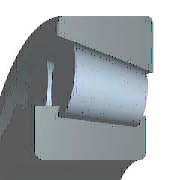
# Autodesk Inventor part: PWTR-0067
Saved by Autodesk Inventor 2021.1 (Build 251245000, 245)
## iProperties
IsCustomPart: 1
Created: 2020-01-21
Part Number: PWTR-0067
Material: Steel, Mild
Description: Taper Roller Bearings Single Row - Precision SKF
Document SubType Name: Modeling
Standard: SKF
Designer: alid
Language: en-US
Size Designation: SKF32004 XC/P5
Categories: <MemberInstance><Categories><Category DisplayName="Shaft Parts" InternalName="7f7aeb1f-a693-4053-b835-cee3144e0d98" Mnemonic="SHFT"><Category DisplayName="Bearings" InternalName="242d30a3-7172-44e6-a363-b0a3d8f1b556" Mnemonic="BRNG"><CategoryParameter DisplayName="Width" InternalName="25fc5f6e-338b-4801-b5ed-8959743e396e" Mnemonic="wdth"/><CategoryParameter DisplayName="Size Designation" InternalName="2c4e891a-c8f4-49ed-a5c1-5131476c6feb" Mnemonic="sizedes"/><CategoryParameter DisplayName="Basic Dynamic Load Rating" InternalName="440972dd-7009-4861-bd45-69ffbb461423" Mnemonic="bdynlrat"/><CategoryParameter DisplayName="Shaft Diameter" InternalName="91302473-2833-4451-a660-c5d4a8d6a031" Mnemonic="shaftdia"/><CategoryParameter DisplayName="Touch Angle" InternalName="aa21a452-7974-4a55-b5cf-1c2972de2aea" Mnemonic="TouchAngle"/><CategoryParameter DisplayName="Outer Diameter" InternalName="d441686c-04bd-4681-b674-94fbc173ec23" Mnemonic="outdia"/><Category DisplayName="Roller Bearings" InternalName="a40a3fd7-d489-4921-9892-cb944902a182" Mnemonic="ROLLBEAR"><CategoryParameter DisplayName="Basic Static Load Rating" InternalName="124ef669-bc53-497e-8b3b-9e9432584ac1" Mnemonic="bstatlrat"/><CategoryParameter DisplayName="Radial Dynamic Load Factor when Fa/Fr &gt; e" InternalName="1feec4eb-3d91-4913-989d-fa96ab069f3d" Mnemonic="raddynfc2"/><CategoryParameter DisplayName="Axial Dynamic Load Factor when Fa/Fr &gt; e" InternalName="200b4357-faba-40fb-9da6-9412c8ddeb78" Mnemonic="axdynfc2"/><CategoryParameter DisplayName="Radius" InternalName="2322b21e-a448-4b16-bf77-0b09a9a1e5fa" Mnemonic="rad"/><CategoryParameter DisplayName="Min. Shaft Diameter" InternalName="27c639de-1f82-42cb-a17a-a84ebe509f1b" Mnemonic="minshaftdia"/><CategoryParameter DisplayName="Limiting Speed Lubrication Grease" InternalName="34ed7782-22cd-44b7-90f2-16a4b10c8234" Mnemonic="lubgrsp"/><CategoryParameter DisplayName="Mass" InternalName="35563771-cdde-4f36-b8ea-a6490dc90073" Mnemonic="mass"/><CategoryParameter DisplayName="Limiting Speed Oil" InternalName="576744bc-a99a-4f12-bf8b-8b83672ef882" Mnemonic="oilspd"/><CategoryParameter DisplayName="Radial Static Load Factor" InternalName="646321f5-f93b-4aec-b962-0341aa1dcfaf" Mnemonic="raddynfc0"/><CategoryParameter DisplayName="Max. Step Fillet Radius" InternalName="890763e8-95b6-457a-9b07-8de657924e40" Mnemonic="maxstprad"/><CategoryParameter DisplayName="Axial Dynamic Load Factor when Fa/Fr &lt;= e" InternalName="b1d498d2-5149-4618-b12c-23a3d5a7c887" Mnemonic="axdynfc1"/><CategoryParameter DisplayName="Radial Dynamic Load Factor when Fa/Fr &lt;= e" InternalName="b75e8b40-fb1d-483d-887b-ce2ffe1b5422" Mnemonic="raddynfc1"/><CategoryParameter DisplayName="Friction Factor" InternalName="ceddb76f-d381-429d-bef5-367584929fdf" Mnemonic="fricfct"/><CategoryParameter DisplayName="Axial Static Load Factor" InternalName="ea413b62-e115-405b-882c-23d570c3be21" Mnemonic="axdynfc0"/><CategoryParameter DisplayName="Limiting Value for Factor Determination" InternalName="f0539972-a230-481a-8ae0-28002199c8fb" Mnemonic="limvalfac"/><CategoryParameter DisplayName="Exponent for Determining Life" InternalName="f80a4cc4-8fb3-4eaa-808e-6f490e608712" Mnemonic="lifeexp"/><CategoryParameter DisplayName="Max. Hub Step Diameter" InternalName="feeea31f-2614-4692-af6e-a054e6e558b2" Mnemonic="maxhubdia"/><Category DisplayName="Tapered Roller Bearings" InternalName="326936b4-87e6-427a-a604-f9fe807308df" Mnemonic="RBTRB"/></Category></Category></Category><Category DisplayName="DataType" InternalName="23b78d0f-2648-40c6-8793-ca6db495c9e8" Mnemonic="DATATYPE"><CategoryParameter DisplayName="DisplayName" InternalName="05415f3d-3907-474b-a020-eb9d644f4cf3" Mnemonic="DISPLAYNAME"/><CategoryParameter DisplayName="Standard" InternalName="0c0a119c-1e12-4c84-803f-101930972f5e" Mnemonic="STANDARD"/><CategoryParameter DisplayName="Description" InternalName="13903e3d-64b1-4950-80da-f627842ea37f" Mnemonic="DESCRIPTION"/><CategoryParameter DisplayName="Designation" InternalName="2675968c-4ce5-49e0-a4f5-552d29089031" Mnemonic="DESIGNATION"/><CategoryParameter DisplayName="Default Row" InternalName="2af9ec52-faaa-4026-b378-f9fa4afca842" Mnemonic="DEFAULTROW"/><CategoryParameter DisplayName="Folder Name" InternalName="3f06958e-8713-4116-9be7-ed6184ecc97b" Mnemonic="FOLDERNAME"/><CategoryParameter DisplayName="Revision Guid" InternalName="45a75005-10b1-4dfc-8d6d-dfe629f0b93c" Mnemonic="REVISIONGUID"/><CategoryParameter DisplayName="FileName" InternalName="8b46a4cc-9585-4fed-90c3-899f57e09a73" Mnemonic="FILENAME"/><CategoryParameter DisplayName="StdsOrg" InternalName="8f5914e1-4693-403f-8ab5-d37768198c9d" Mnemonic="STDSORG"/><CategoryParameter DisplayName="Family Version" InternalName="914462f6-6e19-4b14-ba84-155b9680b1d0" Mnemonic="FAMILYREVISION"/><CategoryParameter DisplayName="Standard Revision" InternalName="91d5a463-65c2-4fde-b823-3b7fea5e8e17" Mnemonic="STANDARDREVISION"/><CategoryParameter DisplayName="Member Revision" InternalName="a65d44b9-392f-4f4f-857b-e4b3d54996fe" Mnemonic="MEMBERREVISION"/><CategoryParameter DisplayName="ClipFormat" InternalName="bc51e27b-3422-4e78-93ef-cec197ddf230" Mnemonic="CLIPFORMAT"/><CategoryParameter DisplayName="Manufacturer" InternalName="cd6c7a72-a28a-4e50-99a9-2c7f4e13e5ad" Mnemonic="MANUFACTURER"/><CategoryParameter DisplayName="InternalName" InternalName="cf1d0246-76d9-4b4a-8305-fa0409afb5c1" Mnemonic="INTERNALNAME"/><CategoryParameter DisplayName="IsMetric" InternalName="e2385c5b-1ea4-4823-96a8-8de651266ec3" Mnemonic="ISMETRIC"/><Category DisplayName="Part" InternalName="c0e0b642-3bcb-4cc8-9e80-f96d35c4afa4" Mnemonic="PART"><CategoryParameter DisplayName="Part Number" InternalName="016b6077-bfbe-49bd-92c9-d8d59c39c941" Mnemonic="PARTNUMBER"/><CategoryParameter DisplayName="Stock Number" InternalName="4dba7c1c-e26c-444e-836c-b08b433409a8" Mnemonic="STOCKNUMBER"/><CategoryParameter DisplayName="Material Key" InternalName="5c9a8adb-dd2b-4535-b97f-0a94a95fe41f" Mnemonic="MATERIALKEY"/><CategoryParameter DisplayName="Material" InternalName="818a152a-d3c3-49ca-80ee-df7d91421b8e" Mnemonic="MATERIAL"/></Category></Category><Category DisplayName="Legacy Map DA" InternalName="924fff40-ddd0-4eff-ad42-30e3774ef79e" Mnemonic="LEGACYMAPDA"><CategoryParameter DisplayName="DACookie" InternalName="316934ee-8fe1-4c7a-9c36-f2d79e1add1a" Mnemonic="DACOOKIE"/></Category><Category DisplayName="LegacyMap" InternalName="cd87c42b-3e48-431e-b5c0-1cbeb14dfe77" Mnemonic="LEGACYMAP"><CategoryParameter DisplayName="unique DA member ID" InternalName="0918ad47-427f-4fed-ae26-24c81c58f590" Mnemonic="DACOOKIE"/><CategoryParameter DisplayName="Merge11 ID" InternalName="0ee8fb18-e2ed-4f39-96f6-1f4b5f50aa71" Mnemonic="MERGE11"/><CategoryParameter DisplayName="unique CC member ID" InternalName="5193edd4-b2b0-4ab4-9d54-de900eee34e0" Mnemonic="CCCOOKIE"/><CategoryParameter DisplayName="Split ID" InternalName="72b5c83c-be7f-45c4-ae51-9160ea6deb26" Mnemonic="SPLIT"/><CategoryParameter DisplayName="MemberID" InternalName="8e5e0294-fc51-4c8f-b3d7-003dc5ed94f6" Mnemonic="MEMBERID"/><CategoryParameter DisplayName="CatalogName" InternalName="d99d1e27-aa94-4de2-af4c-c348882a6f4f" Mnemonic="CATALOGNAME"/><CategoryParameter DisplayName="FamilyNumber" InternalName="e705e1f4-09cb-413e-91f9-551b4188271e" Mnemonic="FAMILYNUMBER"/></Category></Categories><FamilyTemplate Id="N024720"><FamilyTemplateParameters><FamilyTemplateParameter ObjectType="kUserParameterObject" ValueType="xs:integer" Id="1" ObjectReferenceKey="Diam"/><FamilyTemplateParameter ObjectType="kUserParameterObject" ValueType="xs:integer" Id="2" ObjectReferenceKey="DD"/><FamilyTemplateParameter ObjectType="kUserParameterObject" ValueType="xs:double" Id="3" ObjectReferenceKey="B"/><FamilyTemplateParameter ObjectType="kUserParameterObject" ValueType="xs:double" Id="4" ObjectReferenceKey="CC"/><FamilyTemplateParameter ObjectType="kUserParameterObject" ValueType="xs:integer" Id="5" ObjectReferenceKey="ParT"/><FamilyTemplateParameter ObjectType="kUserParameterObject" ValueType="xs:double" Id="6" ObjectReferenceKey="r"/><FamilyTemplateParameter ObjectType="kUserParameterObject" ValueType="xs:integer" Id="8" ObjectReferenceKey="alfa"/><FamilyTemplateParameter ObjectType="kPropertyObject" ValueType="xs:string" Id="100" ObjectReferenceKey="{32853F0F-3444-11d1-9E93-0060B03C1CA6}" SubObjectId="52"/><FamilyTemplateParameter ObjectType="kPropertyObject" ValueType="xs:string" Id="105" ObjectReferenceKey="{32853F0F-3444-11d1-9E93-0060B03C1CA6}" SubObjectId="5"/><FamilyTemplateParameter ObjectType="kPartComponentDefinitionObject" ValueType="xs:string" Id="110" SubObjectId="Material"/></FamilyTemplateParameters></FamilyTemplate><CategoryParameterMap><ParamToTemplateMap><ParamToTemplate CategoryParameter="//CategoryParameter[@InternalName='05415f3d-3907-474b-a020-eb9d644f4cf3']" ConstantValue="SKF- Taper Roller Bearings, Precision"/><ParamToTemplate CategoryParameter="//CategoryParameter[@InternalName='cf1d0246-76d9-4b4a-8305-fa0409afb5c1']" ConstantValue="F84C4950-AFA6-4409-9E95-6F585BEA7148"/><ParamToTemplate CategoryParameter="//CategoryParameter[@InternalName='3f06958e-8713-4116-9be7-ed6184ecc97b']" ConstantValue="SKF - Taper Roller Bearings, Precision"/><ParamToTemplate CategoryParameter="//CategoryParameter[@InternalName='914462f6-6e19-4b14-ba84-155b9680b1d0']" ConstantValue="10"/><ParamToTemplate CategoryParameter="//CategoryParameter[@InternalName='bc51e27b-3422-4e78-93ef-cec197ddf230']" ConstantValue="CF_INVENTOR.STDPARTS"/><ParamToTemplate CategoryParameter="//CategoryParameter[@InternalName='e2385c5b-1ea4-4823-96a8-8de651266ec3']" ConstantValue="true"/><ParamToTemplate CategoryParameter="//CategoryParameter[@InternalName='13903e3d-64b1-4950-80da-f627842ea37f']" ConstantValue="Taper Roller Bearings Single Row - Precision SKF"/><ParamToTemplate CategoryParameter="//CategoryParameter[@InternalName='8f5914e1-4693-403f-8ab5-d37768198c9d']" TemplateParameter="101"/><ParamToTemplate CategoryParameter="//CategoryParameter[@InternalName='0c0a119c-1e12-4c84-803f-101930972f5e']" ConstantValue="SKF"/><ParamToTemplate CategoryParameter="//CategoryParameter[@InternalName='cd6c7a72-a28a-4e50-99a9-2c7f4e13e5ad']" TemplateParameter="104"/><ParamToTemplate CategoryParameter="//CategoryParameter[@InternalName='91d5a463-65c2-4fde-b823-3b7fea5e8e17']" TemplateParameter="103"/><ParamToTemplate CategoryParameter="//CategoryParameter[@InternalName='45a75005-10b1-4dfc-8d6d-dfe629f0b93c']" ConstantValue="35ea33a0-70f2-4056-843a-40b698840a71"/><ParamToTemplate CategoryParameter="//CategoryParameter[@InternalName='2af9ec52-faaa-4026-b378-f9fa4afca842']" ConstantValue="10"/><ParamToTemplate CategoryParameter="//CategoryParameter[@InternalName='8b46a4cc-9585-4fed-90c3-899f57e09a73']" ConstantValue="SKF32004 XC/P5"/><ParamToTemplate CategoryParameter="//CategoryParameter[@InternalName='a65d44b9-392f-4f4f-857b-e4b3d54996fe']" ConstantValue="60633b30-7c0a-4b0a-9e61-588410ecd8ec"/><ParamToTemplate CategoryParameter="//CategoryParameter[@InternalName='124ef669-bc53-497e-8b3b-9e9432584ac1']" ConstantValue="27000"/><ParamToTemplate CategoryParameter="//CategoryParameter[@InternalName='34ed7782-22cd-44b7-90f2-16a4b10c8234']" ConstantValue="8500"/><ParamToTemplate CategoryParameter="//CategoryParameter[@InternalName='ceddb76f-d381-429d-bef5-367584929fdf']" ConstantValue="0.0018"/><ParamToTemplate CategoryParameter="//CategoryParameter[@InternalName='f80a4cc4-8fb3-4eaa-808e-6f490e608712']" ConstantValue="3.33333"/><ParamToTemplate CategoryParameter="//CategoryParameter[@InternalName='27c639de-1f82-42cb-a17a-a84ebe509f1b']" ConstantValue="25"/><ParamToTemplate CategoryParameter="//CategoryParameter[@InternalName='feeea31f-2614-4692-af6e-a054e6e558b2']" ConstantValue="37"/><ParamToTemplate CategoryParameter="//CategoryParameter[@InternalName='890763e8-95b6-457a-9b07-8de657924e40']" ConstantValue="0.6"/><ParamToTemplate CategoryParameter="//CategoryParameter[@InternalName='576744bc-a99a-4f12-bf8b-8b83672ef882']" ConstantValue="12000"/><ParamToTemplate CategoryParameter="//CategoryParameter[@InternalName='f0539972-a230-481a-8ae0-28002199c8fb']" ConstantValue="0.37"/><ParamToTemplate CategoryParameter="//CategoryParameter[@InternalName='646321f5-f93b-4aec-b962-0341aa1dcfaf']" ConstantValue="0.5"/><ParamToTemplate CategoryParameter="//CategoryParameter[@InternalName='ea413b62-e115-405b-882c-23d570c3be21']" ConstantValue="0.9"/><ParamToTemplate CategoryParameter="//CategoryParameter[@InternalName='b75e8b40-fb1d-483d-887b-ce2ffe1b5422']" ConstantValue="1"/><ParamToTemplate CategoryParameter="//CategoryParameter[@InternalName='b1d498d2-5149-4618-b12c-23a3d5a7c887']" ConstantValue="0"/><ParamToTemplate CategoryParameter="//CategoryParameter[@InternalName='2c4e891a-c8f4-49ed-a5c1-5131476c6feb']" ConstantValue="32004 XC/P5"/><ParamToTemplate CategoryParameter="//CategoryParameter[@InternalName='316934ee-8fe1-4c7a-9c36-f2d79e1add1a']" ConstantValue="*ISO~N024720A~SKF 32004 XC/P5*AFN~N024720A~SKF 32004 XC/P5*ANS~N024720A~SKF 32004 XC/P5*"/><ParamToTemplate CategoryParameter="//CategoryParameter[@InternalName='0918ad47-427f-4fed-ae26-24c81c58f590']" ConstantValue="*ISO~N024720A~SKF 32004 XC/P5*AFN~N024720A~SKF 32004 XC/P5*ANS~N024720A~SKF 32004 XC/P5*"/><ParamToTemplate CategoryParameter="//CategoryParameter[@InternalName='0ee8fb18-e2ed-4f39-96f6-1f4b5f50aa71']" ConstantValue="^1FF598A5-DCBF-4D03-99DD-51C67A5B1954^3ADC193E-2142-431A-9EEA-E87C8E0B94A1^36F4839B-D4FF-4949-8334-EE9110708ED8^"/><ParamToTemplate CategoryParameter="//CategoryParameter[@InternalName='25fc5f6e-338b-4801-b5ed-8959743e396e']" TemplateParameter="3"/><ParamToTemplate CategoryParameter="//CategoryParameter[@InternalName='d441686c-04bd-4681-b674-94fbc173ec23']" TemplateParameter="2"/><ParamToTemplate CategoryParameter="//CategoryParameter[@InternalName='2675968c-4ce5-49e0-a4f5-552d29089031']" TemplateParameter="100"/><ParamToTemplate CategoryParameter="//CategoryParameter[@InternalName='91302473-2833-4451-a660-c5d4a8d6a031']" TemplateParameter="1"/><ParamToTemplate CategoryParameter="//CategoryParameter[@InternalName='818a152a-d3c3-49ca-80ee-df7d91421b8e']" TemplateParameter="110"/><ParamToTemplate CategoryParameter="//CategoryParameter[@InternalName='016b6077-bfbe-49bd-92c9-d8d59c39c941']" TemplateParameter="105"/><ParamToTemplate CategoryParameter="//CategoryParameter[@InternalName='2322b21e-a448-4b16-bf77-0b09a9a1e5fa']" TemplateParameter="6"/></ParamToTemplateMap></CategoryParameterMap></MemberInstance>
Density: 7.85 g/cm^3
Appearance: Semi-Polished
Stock Number: SKF32004 XC/P5
Author: alid
Revision Number: A
Autodesk Inventor part; units mm, degrees
ref_plane "WorkPlane4" through (0, 0, 0) normal (0, 0, 1) x (1, 0, 0)
ref_plane "WorkPlane1" through (0, 0, 0) normal (0, 0, 1) x (1, 0, 0)
ref_plane "Work Plane3" through (0, 0, -15) normal (0, 0, 1) x (1, 0, 0)
ref_plane "WorkPlane2" through (0, 0, 15) normal (0, 0, 1) x (1, 0, 0)
sketch "Sketch1" plane through (0, 0, 0) normal (0, 0, 1) x (1, 0, 0)
  point P0 (0, 0)
sketch "Sketch2" plane through (0, 0, 15) normal (0, 0, 1) x (1, 0, 0)
  point P0 (0, 0)
sketch "Sketch3" plane through (0, 0, 0) normal (0, 0, 1) x (1, 0, 0)
  circle A0 centre (0, 0) radius 15.5
  dimension "d2" = 31
extrude "Extrusion1" add sketch "Sketch3" along normal blind 15
sketch "Sketch4" plane through (0, 0, 15) normal (0, 0, 1) x (1, 0, 0)
  circle A0 centre (0, 0) radius 15.5 projected
hole "Hole1" at (0, 0, 15) direction (0, 0, -1) diameter 20 end through all
sketch "Sketch5" plane through (0, 0, 0) normal (1, 0, 0) x (0, 1, 0)
  line L0 (16.471593, 15) -> (14.125, 15)
  line L1 (14.125, 15) -> (14.125, 11.985238)
  line L2 (12.066474, 11.547685) -> (14.125, 11.985238)
  line L3 (12.066474, 11.547685) -> (13.433526, 2.283254)
  line L4 (13.433526, 2.283254) -> (16.471593, 2.929015)
  line L5 (16.471593, 15) -> (16.471593, 2.929015)
  line L6 (12.75, 6.915469) -> (15.5, 7.5) construction
  line L7 (14.072762, 14.214627) -> (17.032483, 0.290235) construction
  line L8 (0, 15.438993) -> (0, -16.363725) construction
  line L9 (-15.5, 15) -> (15.5, 15) construction
  line L10 (-15.5, 0) -> (15.5, 0) construction
  line L11 (0, 29.363727) -> (0, -16.363727)
  line L12 (0, -25.509217) -> (0, 38.509217)
  dimension "d14" = 12
  dimension "d17" = 9.26443
  dimension "d37" = 31
  dimension "d42" = 4.63222
  dimension "d49" = 3.60606
  dimension "d54" = 7.5
  dimension "d55" = 2.75
  dimension "d56" = 28.25
  constraints: 20 end point, 3 collinear, 3 parallel, 2 perpendicular, 2 point on line, 2 vertical, 1 horizontal, 1 midpoint
  measures "d14" angle of L8 L7
  measures "d17" vertical distance of L2.start L3.end
  measures "d37" diameter of L6.end L11
  measures "d42" vertical distance of L3.end L6.start
  measures "d49" angle of L7 L3
  measures "d54" distance from line of L10 L6.end
  measures "d55" horizontal distance of L6.start L6.end
  measures "d56" diameter of L0.end L12
revolve "Revolution1" cut sketch "Sketch5" angle 360 about axis through (0, 0, 29.363727) along (0, 0, -1)
sketch "Sketch6" plane through (0, 0, 0) normal (1, 0, 0) x (0, 1, 0)
  line L0 (13.433526, 2.283254) -> (16.471593, 2.929015)
  line L1 (13.433526, 2.283254) -> (12.066474, 11.547685)
  line L2 (12.066474, 11.547685) -> (14.528407, 12.070985)
  line L3 (16.471593, 2.929015) -> (14.528407, 12.070985)
  line L4 (13.8641, 15.196307) -> (16.925604, 0.793058) construction
  line L5 (12.75, 6.915469) -> (15.5, 7.5) construction
  line L6 (0, 29.363728) -> (0, -16.363726) construction
  line L7 (-15.5, 0) -> (15.5, 0) construction
  line L8 (16.471593, 2.929015) -> (14.528407, 12.070985)
  line L9 (0, -25.509216) -> (0, 38.509219)
  line L10 (13.433526, 2.283254) -> (12.066474, 11.547685)
  line L11 (15.5, 2.722497) -> (13.433526, 2.283254)
  line L12 (12.066474, 11.547685) -> (14.125, 11.985238)
  dimension "d20" = 12
  dimension "d23" = 4.63222
  dimension "d46" = 31
  dimension "d47" = 9.26443
  constraints: 17 end point, 3 point on line, 2 collinear, 2 midpoint, 2 parallel, 1 perpendicular
  measures "d20" angle of L6 L4
  measures "d23" vertical distance of L5.start L0.start
  measures "d46" diameter of L5.end L6
  measures "d47" vertical distance of L0.start L1.end
revolve "Revolution2" add sketch "Sketch6" angle 360 about axis through (0, 16.471593, 2.929015) along (0, -0.2079117, 0.9781476)
pattern_circular "PolarArray1" count 11 over 360 about axis through (0, 0, 0) along (0, 0, 1) of "Revolution2"
sketch "Sketch7" plane through (0, 0, 0) normal (1, 0, 0) x (0, 1, 0)
  line L0 (21, 3) -> (19.67031, 3)
  line L1 (21, 15) -> (21, 3)
  line L2 (16.318482, 15) -> (21, 15)
  line L3 (19.67031, 3) -> (16.318482, 15)
  line L4 (-15.5, 0) -> (15.5, 0) construction
  line L5 (0, 29.363727) -> (0, -16.363727) construction
  line L6 (0, 29.363727) -> (0, -16.363727)
  line L7 (0, -25.509217) -> (0, 38.509217)
  line L8 (19.50966, 3.574777) -> (16.99034, 12.594285)
  line L9 (14.125, 15) -> (-14.125, 15)
  dimension "d29" = 12
  dimension "d44" = 42
  dimension "d45" = 15
  dimension "d63" = 0.0001
  constraints: 12 end point, 2 horizontal, 1 collinear, 1 parallel, 1 vertical
  measures "d29" distance of L1.start L0.start
  measures "d44" diameter of L1 L5
  measures "d45" distance between parallel lines of L4 L2
  measures "d63" distance between parallel lines of L3 L8
fillet "Fillet1" radius 0.6 1 edges at (0, 10, 0)
fillet "Fillet2" radius 0.6 1 edges at (0, 10, 15)
revolve "Revolution3" add sketch "Sketch7" angle 360 about axis through (0, 0, 29.363727) along (0, 0, -1)
equation "\"d6\" = Diam"
equation "\"d29\" = CC"
equation "\"d44\" = DD"
equation "\"d45\" = ParT"
equation "\"d34\" = r"
equation "\"d3\" = B"
equation "\"d33\" = r"
equation "\"d2\" = msp_dd2"
equation "\"d37\" = msp_mdtds"
equation "\"d42\" = d23"
equation "\"d49\" = msp_ang"
equation "\"d54\" = 0.5 * ParT"
equation "\"d55\" = 0.5 * msp_dd0"
equation "\"d56\" = msp_mdtds - 0.5 * msp_dd0"
equation "\"d46\" = d37"
equation "\"d47\" = d17"
equation "\"B\" = 15"
equation "\"DD\" = 42"
equation "\"Diam\" = 20"
equation "\"msp_dd2\" = 0.5 * Diam + 0.5 * DD"
equation "\"ParT\" = 15"
equation "\"r\" = 0.6"
equation "\"CC\" = 12"
equation "\"msp_dd0\" = -0.25 * Diam + 0.25 * DD"
equation "\"msp_mdtds\" = 0.5 * Diam + 0.5 * DD"
equation "\"msp_l0\" = 0.8 * CC"
equation "\"msp_pom2\" = alfa + msp_ang"
equation "\"msp_ang\" = 3.606059deg"
equation "\"alfa\" = 12"
body "Solid1"
